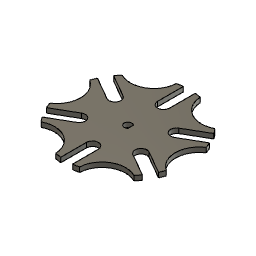
2.DrivenWheel (Autodesk Fusion 360 design; units mm, degrees)
Autodesk Fusion 360 part; units mm, degrees
sketch "Sketch1" plane through (0, 0, 0) normal (0, 1, 0) x (1, 0, 0)
  line L0 (36.5192, 19.3301) -> (17.7088, 30.1903)
  line L1 (12.7088, 21.5301) -> (31.5192, 10.6699)
  arc A0 (31.5192, 10.6699) -> (36.5192, 19.3301) centre (34.0192, 15) ccw
  arc A1 (10.8333, -16.8119) -> (10.8333, 16.8119) centre (0, 0) ccw
  arc A2 (31.5192, 10.6699) -> (36.5192, 19.3301) centre (34.0192, 15) ccw
  arc A3 (12.7088, 21.5301) -> (10.8333, 16.8119) centre (60, 0) ccw
  line L2 (31.5192, -10.6699) -> (12.7088, -21.5301)
  arc A4 (36.5192, -19.3301) -> (31.5192, -10.6699) centre (34.0192, -15) ccw
  line L3 (17.7088, -30.1903) -> (36.5192, -19.3301)
  arc A5 (49.9762, -50.9855) -> (20.8572, -34.1736) centre (30, -51.9615) ccw
  line L4 (55, -30) -> (55, -51.7204)
  arc A6 (65, -30) -> (55, -30) centre (60, -30) ccw
  line L5 (65, -51.7204) -> (65, -30)
  arc A7 (99.1428, -34.1736) -> (70.0238, -50.9855) centre (90, -51.9615) ccw
  line L6 (83.4807, -19.3301) -> (102.2911, -30.1903)
  arc A8 (88.4807, -10.6699) -> (83.4807, -19.3301) centre (85.9807, -15) ccw
  line L7 (107.2911, -21.5301) -> (88.4807, -10.6699)
  arc A9 (109.1666, 16.8119) -> (109.1666, -16.8119) centre (120, 0) ccw
  line L8 (88.4807, 10.6699) -> (107.2911, 21.5301)
  arc A10 (83.4807, 19.3301) -> (88.4807, 10.6699) centre (85.9807, 15) ccw
  line L9 (102.2911, 30.1903) -> (83.4807, 19.3301)
  arc A11 (70.0238, 50.9855) -> (99.1428, 34.1736) centre (90, 51.9615) ccw
  line L10 (65, 30) -> (65, 51.7204)
  arc A12 (55, 30) -> (65, 30) centre (60, 30) ccw
  line L11 (55, 51.7204) -> (55, 30)
  arc A13 (20.8572, 34.1736) -> (49.9762, 50.9855) centre (30, 51.9615) ccw
  arc A14 (55, 51.7204) -> (49.9762, 50.9855) centre (60, 0) ccw
  arc A15 (20.8572, 34.1736) -> (17.7054, 30.1856) centre (60, 0) ccw
  arc A16 (70.0238, 50.9855) -> (65, 51.7204) centre (60, 0) ccw
  arc A17 (102.2911, 30.1903) -> (99.1428, 34.1736) centre (60, 0) ccw
  arc A18 (109.1666, 16.8119) -> (107.2911, 21.5301) centre (60, 0) ccw
  arc A19 (107.2911, -21.5301) -> (109.1666, -16.8119) centre (60, 0) ccw
  arc A20 (99.1428, -34.1736) -> (102.2911, -30.1903) centre (60, 0) ccw
  arc A21 (65, -51.7204) -> (70.0238, -50.9855) centre (60, 0) ccw
  arc A22 (49.9762, -50.9855) -> (55, -51.7204) centre (60, 0) ccw
  arc A23 (10.8333, -16.8119) -> (12.7088, -21.5301) centre (60, 0) ccw
  arc A24 (17.7088, -30.1903) -> (20.8572, -34.1736) centre (60, 0) ccw
  line L12 (60, 0) -> (62.25, 0)
  line L13 (62.25, 2.3452) -> (62.25, -2.3452)
  arc A25 (62.25, 2.3452) -> (62.25, -2.3452) centre (60, 0) ccw
  dimension "d5" = 360
  constraint tangent L1 A0
  constraint tangent L0 A0
  constraint parallel L0 L1
  constraint concentric A0 A2
  constraint coincident A1.centre origin
  constraint concentric A3 A23
  constraint coincident L0.end A23
  constraint concentric A14 A23
  constraint concentric A14 A15
  constraint concentric A16 A23
  constraint concentric A17 A23
  constraint concentric A18 A23
  constraint concentric A19 A23
  constraint concentric A20 A23
  constraint concentric A21 A23
  constraint concentric A22 A23
  constraint concentric A23 A24
  constraint concentric A24 A25
  constraint coincident A3.centre A14.centre
  constraint horizontal L12
  constraint perpendicular L12 L13
extrude "Extrude1" add sketch "Sketch1" along normal blind 4
